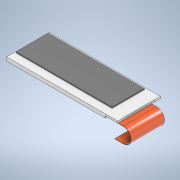
# Autodesk Inventor part: display
Saved by Autodesk Inventor 2020 (Build 240168000, 168)
## iProperties
Created: 2022-02-28
Part Number: display
Material: Типовые
Document SubType Name: Modeling
Designer: NoName
Density: 1 g/cm^3
Appearance: По умолчанию
Author: NoName
Autodesk Inventor part; units mm, degrees
ref_plane "YZ Plane" through (0, 0, 0) normal (1, 0, 0) x (0, 1, 0)
ref_plane "XZ Plane" through (0, 0, 0) normal (0, 1, 0) x (-1, 0, 0)
ref_plane "XY Plane" through (0, 0, 0) normal (0, 0, 1) x (1, 0, 0)
sketch "Эскиз8" plane through (0, 0, 0) normal (0, 1, 0) x (-1, 0, 0)
  line L0 (0, 0) -> (-26.6, 0)
  line L1 (-26.6, 0) -> (-26.6, -11.5)
  line L2 (-26.6, -11.5) -> (0, -11.5)
  line L3 (0, -11.5) -> (0, 0)
  dimension "d18" = 11.5
  dimension "d19" = 26.6
  constraints: 8 end point, 2 parallel, 1 horizontal, 1 perpendicular
  measures "d18" distance between parallel lines of L0 L2
  measures "d19" distance between parallel lines of L1 L3
extrude "Выдавливание4" add sketch "Эскиз8" along normal blind 0.5
sketch "Эскиз9" plane through (0, 0.5, 0) normal (0, 1, 0) x (1, 0, 0)
  line L0 (0, 0) -> (26.6, 0) projected
  line L1 (0, 0) -> (30, 0)
  line L2 (30, 0) -> (30, 11.5)
  line L3 (30, 11.5) -> (0, 11.5)
  line L4 (0, 11.5) -> (0, 0)
  dimension "d22" = 30
  constraints: 8 end point, 2 parallel, 1 horizontal, 1 perpendicular
  measures "d22" distance between parallel lines of L4 L2
extrude "Выдавливание5" add sketch "Эскиз9" along normal blind 0.5
sketch "Эскиз10" plane through (0, 1, 0) normal (0, 1, 0) x (1, 0, 0)
  line L0 (0.35, 2.2) -> (26.25, 2.2)
  line L1 (26.25, 2.2) -> (26.25, 11)
  line L2 (26.25, 11) -> (0.35, 11)
  line L3 (0.35, 11) -> (0.35, 2.2)
  line L4 (30, 11.5) -> (0, 11.5) projected
  line L5 (0, 11.5) -> (0, 0) projected
  dimension "d25" = 25.9
  dimension "d26" = 8.8
  dimension "d27" = 0.5
  dimension "d28" = 0.35
  constraints: 8 end point, 2 parallel, 1 horizontal, 1 perpendicular
  measures "d25" distance between parallel lines of L1 L3
  measures "d26" distance between parallel lines of L0 L2
  measures "d27" distance between parallel lines of L4 L2
  measures "d28" distance between parallel lines of L5 L3
extrude "Выдавливание6" add sketch "Эскиз10" along normal blind 0.2
ref_plane "РабПлоскость2" through (0, 0, -0.1) normal (0, 0, 1) x (1, 0, 0)
sketch "Эскиз12" plane through (0, 0, -0.1) normal (0, 0, 1) x (1, 0, 0)
  arc A0 (31.4, -3.6) -> (31.4, 0.4) centre (31.4, -1.6) ccw
  arc A1 (31.4, -3.7) -> (31.4, 0.5) centre (31.4, -1.6) ccw
  line L0 (31.4, 0.4) -> (27.6, 0.4)
  line L1 (27.6, 0.4) -> (27.6, 0.5)
  line L2 (31.4, 0.5) -> (27.6, 0.5)
  line L3 (30, 0.5) -> (30, 1) projected
  line L4 (26.6, 0.5) -> (30, 0.5) projected
  line L5 (26.6, 0) -> (26.6, 0.5) projected
  line L6 (31.4, -3.7) -> (29.08, -3.7)
  line L7 (29.08, -3.7) -> (29.08, -3.6)
  line L8 (29.08, -3.6) -> (31.4, -3.6)
  point P0 (0, 0)
  dimension "d34" = 0.1
  dimension "d36" = 1.4
  dimension "d37" = 1
  dimension "d38" = 2
  dimension "d39" = 2.32
  constraints: 12 end point, 4 perpendicular, 4 point on circle, 4 vertical alignment, 2 centre point, 2 horizontal, 1 coincident, 1 point on line
  measures "d34" radial gap between concentric circles of A1 A0
  measures "d36" distance from line of L3 A0.centre
  measures "d37" distance between parallel lines of L5 L1
  measures "d38" radius of A0
  measures "d39" distance of L6.start L6.end
extrude "Выдавливание7" add sketch "Эскиз12" against normal blind 9
